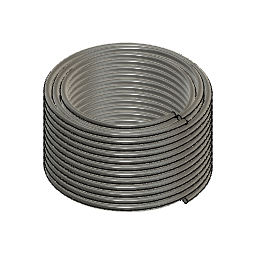
cabo cftv (Autodesk Fusion 360 design; units mm, degrees)
Autodesk Fusion 360 part; units mm, degrees
note: some values were not read from the file. Chosen so that the rebuilt part matches the saved one: the hand of a thread or coil.
sketch "Sketch1" plane through (0, 0, 0) normal (0, 0, 1) x (1, 0, 0)
coil "CoilPrimitive1" add diameter 400 section circle size 20 on centre turns 12 pitch 25 right hand placed x (1, 0, 0) y (0, 1, 0) z (0, 0, 1) at (0, 0, 0) makes body 1
coil "CoilPrimitive2" add diameter 450 section circle size 20 on centre turns 12 pitch 25 left hand placed x (1, 0, 0) y (0, 1, 0) z (0, 0, 1) at (0, 0, 0) separate body makes body 2
coil "CoilPrimitive3" add diameter 500 section circle size 20 on centre turns 12 pitch 25 right hand placed x (1, 0, 0) y (0, 1, 0) z (0, 0, 1) at (0, 0, 0) separate body makes body 3
